Autodesk Fusion 360 part; units mm, degrees
(part 2 of 5)
sketch "Sketch1" plane through (0, 0, 0) normal (0, 0, 1) x (1, 0, 0)
  line L0 (-30.55, 69.6) -> (-28.55, 69.6)
  line L1 (-28.55, 69.6) -> (-28.55, 0)
  line L2 (-28.55, 0) -> (-30.55, 0)
  line L3 (-30.55, 0) -> (-30.55, 69.6)
  line L4 (28.55, 69.6) -> (30.55, 69.6)
  line L5 (30.55, 69.6) -> (30.55, 0)
  line L6 (30.55, 0) -> (28.55, 0)
  line L7 (28.55, 0) -> (28.55, 69.6)
  dimension "d1" = 69.6
  dimension "d2" = 69.6
  dimension "d3" = 2
  dimension "d4" = 2
  dimension "d5" = 57.1
  dimension "d6" = 28.55
  constraint horizontal L0
  constraint vertical L1
  constraint horizontal L2
  constraint vertical L3
  constraint horizontal L4
  constraint vertical L5
  constraint horizontal L6
  constraint vertical L7
  constraint horizontal L0.start L4.start
  constraint horizontal origin L1.end
  measures "d1" distance of L0 L2
  measures "d2" distance of L4 L6
  measures "d3" distance of L1 L3
  measures "d4" distance of L5 L7
  measures "d5" distance of L1 L7
  measures "d6" distance of origin L7
extrude "Extrude1" add sketch "Sketch1" along normal blind 20 makes body 1 at (-28.55, 46.4, 6.6667) makes body 2 at (30.55, 46.4, 6.6667)
sketch "Sketch3" plane through (0, 0, 20) normal (0, 0, 1) x (-1, 0, 0)
  line L0 (-28.55, 0) -> (-30.55, 0)
  line L1 (-30.55, 0) -> (-30.55, -69.6)
  line L2 (-30.55, -69.6) -> (-28.55, -69.6)
  line L3 (-28.55, -69.6) -> (-28.55, 0)
  arc A0 (-28.55, -69.6) -> (28.55, -69.6) centre (0, 38.699) ccw
  arc A1 (-30.55, -71.6) -> (30.55, -71.6) centre (0, 52.672) ccw
  line L4 (30.55, -71.6) -> (30.55, -69.6)
  line L5 (-30.55, -71.6) -> (-30.55, -69.6)
  line L6 (-28.55, -69.6) -> (-30.55, -69.6)
  line L7 (28.55, -69.6) -> (30.55, -69.6)
  point P0 (-28.55, -69.6)
  point P1 (28.55, -69.6)
  point P2 (0, -73.3)
  point P3 (0, -75.3)
  point P4 (30.55, -71.6)
  point P5 (-30.55, -71.6)
  point P6 (30.55, -69.6)
  dimension "d9" = 3.7
  dimension "d10" = 2
  dimension "d11" = 2
  dimension "d12" = 2
  constraint coincident P0 L2.end
  constraint coincident P2 A0
  constraint coincident P1 A0.end
  constraint vertical origin P2
  constraint vertical P2 P3
  constraint vertical L1.end P5
  constraint vertical P4 P6
  constraint coincident P3 A1
  constraint coincident P5 A1.start
  constraint coincident P4 A1.end
  constraint coincident P6 L4.end
  constraint coincident L1.end L2.start
  measures "d9" vertical distance of P0 P2
  measures "d10" distance of P2 P3
  measures "d11" distance of P4 P6
  measures "d12" distance of L1.end P5
extrude "Extrude2" add sketch "Sketch3" against normal blind 20 contours L2 A0 A1 L4 L5 L6 L7 bodies 1 2
sketch "Sketch4" plane through (30.55, 0, 0) normal (1, 0, 0) x (0, 1, 0)
  line L0 (0, 0) -> (71.6, 0)
  line L1 (71.6, 0) -> (71.6, 20)
  line L2 (71.6, 20) -> (0, 20)
  line L3 (0, 20) -> (0, 0)
  line L4 (0, 0) -> (20, 0)
  line L5 (20, 0) -> (20, -4)
  line L6 (20, -4) -> (0, -4)
  line L7 (0, -4) -> (0, 0)
  dimension "d15" = 4
  dimension "d16" = 20
  constraint horizontal L4
  constraint vertical L5
  constraint horizontal L6
  constraint vertical L7
  constraint coincident L0.start L3.end
  measures "d15" distance of L4 L6
  measures "d16" distance of L5 L7
extrude "Extrude3" add sketch "Sketch4" against normal blind 2 contours L0 L4 L5 L6 L7 bodies 1
sketch "Sketch5" plane through (-30.55, 0, 0) normal (-1, 0, 0) x (0, -1, 0)
  line L0 (-71.6, 0) -> (0, 0)
  line L1 (0, 0) -> (0, 20)
  line L2 (0, 20) -> (-71.6, 20)
  line L3 (-71.6, 20) -> (-71.6, 0)
  line L4 (0, 0) -> (-20, 0)
  line L5 (-20, 0) -> (-20, -4)
  line L6 (-20, -4) -> (0, -4)
  line L7 (0, -4) -> (0, 0)
  dimension "d19" = 4
  dimension "d20" = 20
  constraint horizontal L4
  constraint vertical L5
  constraint horizontal L6
  constraint vertical L7
  constraint coincident L0.end L1.start
  measures "d19" distance of L4 L6
  measures "d20" distance of L5 L7
extrude "Extrude4" add sketch "Sketch5" against normal blind 2 contours L0 L4 L5 L6 L7 bodies 1
fillet "Fillet2" radius 2 4 edges at (30.55, 71.6, 10) (-30.55, 71.6, 10) (29.55, 20, 0) (-29.55, 20, 0) on bodies 1
sketch "Sketch8" plane through (0, 0, 0) normal (0, -1, 0) x (1, 0, 0)
  line L0 (30.55, -4) -> (30.55, 20)
  line L1 (30.55, 20) -> (28.55, 20)
  line L2 (28.55, 20) -> (28.55, -4)
  line L3 (30.55, 20) -> (28.55, 20)
  line L4 (30.55, 36.5) -> (30.55, 20)
  line L5 (-30.55, 20) -> (-28.55, 20)
  line L6 (-30.55, 36.5) -> (-30.55, 20)
  line L7 (28.55, 20) -> (-28.55, 20)
  line L8 (-19.3, 36.5) -> (-19.3, 34.25)
  line L9 (-24.3, 29.25) -> (-26.05, 29.25)
  line L10 (19.3, 36.5) -> (19.3, 34.25)
  line L11 (24.3, 29.25) -> (26.05, 29.25)
  line L12 (-28.55, 26.75) -> (-28.55, 20)
  line L13 (28.55, 26.75) -> (28.55, 20)
  line L14 (-28.05, 39) -> (-21.8, 39)
  line L15 (21.8, 39) -> (28.05, 39)
  arc A0 (30.55, 36.5) -> (28.05, 39) centre (28.05, 36.5) ccw
  arc A1 (-28.05, 39) -> (-30.55, 36.5) centre (-28.05, 36.5) ccw
  arc A2 (21.8, 39) -> (19.3, 36.5) centre (21.8, 36.5) ccw
  arc A3 (28.55, 26.75) -> (26.05, 29.25) centre (26.05, 26.75) ccw
  arc A4 (-26.05, 29.25) -> (-28.55, 26.75) centre (-26.05, 26.75) ccw
  arc A5 (-19.3, 36.5) -> (-21.8, 39) centre (-21.8, 36.5) ccw
  arc A6 (19.3, 34.25) -> (24.3, 29.25) centre (24.3, 34.25) ccw
  arc A7 (-24.3, 29.25) -> (-19.3, 34.25) centre (-24.3, 34.25) ccw
  line L16 (28.55, -4) -> (30.55, -4)
  point P0 (-30.55, 39)
  point P1 (-19.3, 39)
  point P2 (-19.3, 29.25)
  point P3 (-28.55, 29.25)
  point P4 (19.3, 39)
  point P5 (19.3, 29.25)
  point P6 (28.55, 29.25)
  dimension "d41" = 61.1
  dimension "d51" = 9.75
  dimension "d52" = 9.75
  dimension "d53" = 9.25
  dimension "d54" = 9.25
  dimension "d55" = 11.25
  dimension "d56" = 9.25
  dimension "d57" = 2.5
  dimension "d58" = 2.5
  dimension "d59" = 5
  constraint horizontal L3
  constraint vertical L4
  constraint coincident L0.end L1.start
  constraint horizontal L5
  constraint vertical L6
  constraint horizontal L0.end L5.start
  constraint vertical L8
  constraint horizontal L9
  constraint vertical L10
  constraint horizontal L11
  constraint perpendicular L7 L12
  constraint coincident L1.end L2.start
  constraint perpendicular L3 L13
  constraint perpendicular L8 L14
  constraint horizontal P2 P5
  constraint tangent L15 A0
  constraint tangent L4 A0
  constraint coincident P0 L14
  constraint coincident P0 L6
  constraint tangent L14 A1
  constraint tangent L6 A1
  constraint equal A0 A1
  constraint coincident P4 L10
  constraint coincident P4 L15
  constraint tangent L10 A2
  constraint tangent L15 A2
  constraint coincident P6 L11
  constraint coincident P6 L13
  constraint tangent L11 A3
  constraint tangent L13 A3
  constraint equal A2 A3
  constraint coincident P3 L9
  constraint coincident P3 L12
  constraint tangent L9 A4
  constraint tangent L12 A4
  constraint equal A2 A4
  constraint coincident P1 L8
  constraint coincident P1 L14
  constraint tangent L8 A5
  constraint tangent L14 A5
  constraint equal A2 A5
  constraint coincident P5 L11
  constraint coincident P5 L10
  constraint tangent L11 A6
  constraint tangent L10 A6
  constraint coincident P2 L9
  constraint coincident P2 L8
  constraint tangent L9 A7
  constraint tangent L8 A7
  constraint equal A6 A7
  measures "d41" distance of L0.end L5.start
  measures "d51" distance of P1 P2
  measures "d52" distance of P4 P5
  measures "d53" distance of P2 P3
  measures "d54" distance of P5 P6
  measures "d55" distance of P0 P1
  measures "d56" distance of P6 L1.end
  measures "d57" radius of A0
  measures "d58" radius of A2
  measures "d59" radius of A6
extrude "Extrude6" add sketch "Sketch8" against normal blind 20 contours L1 L3 L4 L10 L11 L13 L15 A0 A2 A3 A6 | L5 L6 L8 L9 L12 L14 A1 A4 A5 A7 bodies 1
sketch "Sketch9" plane through (0, 20, 0) normal (0, 1, 0) x (-1, 0, 0)
  arc A0 (-19.3, 36.5) -> (-21.8, 39) centre (-21.8, 36.5) ccw
  line L0 (-21.8, 39) -> (-28.05, 39)
  arc A1 (-28.05, 39) -> (-30.55, 36.5) centre (-28.05, 36.5) ccw
  line L1 (-30.55, 36.5) -> (-30.55, 20)
  line L2 (-30.55, 20) -> (-28.55, 20)
  line L3 (-28.55, 20) -> (-28.55, 26.75)
  arc A2 (-26.05, 29.25) -> (-28.55, 26.75) centre (-26.05, 26.75) ccw
  line L4 (-26.05, 29.25) -> (-24.3, 29.25)
  arc A3 (-24.3, 29.25) -> (-19.3, 34.25) centre (-24.3, 34.25) ccw
  line L5 (-19.3, 34.25) -> (-19.3, 36.5)
  line L6 (30.55, 20) -> (30.55, 36.5)
  point P0 (-24.05, 34.05)
  point P1 (24.05, 34.05)
  dimension "d62" = 6.5
  dimension "d63" = 6.5
  dimension "d64" = 4.95
  constraint horizontal P0 P1
  measures "d62" distance of L1 P0
  measures "d63" distance of P1 L6
  measures "d64" distance of L0 P0
hole "Hole3" at (24.05, 20, 34.05) at (-24.05, 20, 34.05) direction (0, -1, 0) diameter 6.5 depth 12.5 tip angle 180 bodies 1
sketch "Sketch10" plane through (0, 7.5, 0) normal (0, 1, 0) x (-1, 0, 0)
  circle A0 centre (-24.05, 34.05) radius 3.25
  line L0 (-30.55, 36.5) -> (-30.55, 20)
  line L1 (30.55, 20) -> (30.55, 36.5)
  line L2 (-21.8, 39) -> (-28.05, 39)
  point P0 (-24.05, 34.05)
  point P1 (24.05, 34.05)
  dimension "d73" = 6.5
  dimension "d74" = 6.5
  dimension "d75" = 4.95
  constraint horizontal P0 P1
  measures "d73" distance of P0 L0
  measures "d74" distance of P1 L1
  measures "d75" distance of P0 L2
hole "Hole4" at (24.05, 7.5, 34.05) at (-24.05, 7.5, 34.05) direction (0, -1, 0) diameter 3.6 end through all counterbore diameter 6.5 counterbore depth 3 bodies 1
sketch "Sketch11" plane through (30.55, 0, 0) normal (1, 0, 0) x (0, 1, 0)
  line L0 (70.0221, 0) -> (70.0221, 20)
  line L1 (70.0221, 20) -> (20, 20)
  line L2 (20, 20) -> (20, 36.5)
  line L3 (20, 36.5) -> (0, 36.5)
  line L4 (0, 36.5) -> (0, -4)
  line L5 (20, -4) -> (20, -2)
  arc A0 (22, 0) -> (20, -2) centre (22, -2) ccw
  line L6 (22, 0) -> (70.0221, 0)
  arc A1 (8.659, 9.478) -> (8.6579, 10.5518) centre (7.8148, 10.014) ccw
  line L7 (8.659, 9.478) -> (3.8443, 1.8949)
  line L8 (3.8432, 18.1005) -> (8.6579, 10.5518)
  line L9 (0.0001, 36.7902) -> (0.0001, -5.2598)
  arc A2 (3.8432, 18.1005) -> (2.0001, 17.5628) centre (3.0001, 17.5628) ccw
  arc A3 (2.0001, 2.4309) -> (3.8443, 1.8949) centre (3.0001, 2.4309) ccw
  arc A4 (18.0001, 17.5628) -> (16.157, 18.1005) centre (17.0001, 17.5628) ccw
  line L10 (16.088, 20.7084) -> (10.853, 12.3732)
  line L11 (9.1559, 12.3786) -> (3.9952, 20.7138)
  line L12 (3.99, -0.735) -> (9.1549, 7.6441)
  line L13 (15.2412, 22.2402) -> (4.8454, 22.2402)
  line L14 (2.0001, 17.5628) -> (2.0001, 2.4309)
  arc A5 (10.8541, 7.6495) -> (9.1549, 7.6441) centre (10.0062, 7.1193) ccw
  line L15 (20.0001, 40.5402) -> (0.0001, 40.5402)
  arc A6 (3.99, -0.735) -> (4.8412, -2.2598) centre (4.8412, -1.2598) ccw
  line L16 (20.0001, 36.7902) -> (0.0001, 36.7902)
  arc A7 (4.8454, 22.2402) -> (3.9952, 20.7138) centre (4.8454, 21.2402) ccw
  line L17 (15.2454, -2.2598) -> (4.8412, -2.2598)
  line L18 (18.0001, 17.5628) -> (18.0001, 2.4309)
  arc A8 (16.088, 20.7084) -> (15.2412, 22.2402) centre (15.2412, 21.2402) ccw
  line L19 (16.1559, 1.8949) -> (11.3412, 9.478)
  arc A9 (9.1559, 12.3786) -> (10.853, 12.3732) centre (10.0062, 12.9051) ccw
  line L20 (10.8541, 7.6495) -> (16.0933, -0.7296)
  line L21 (11.3423, 10.5518) -> (16.157, 18.1005)
  arc A10 (11.3423, 10.5518) -> (11.3412, 9.478) centre (12.1854, 10.014) ccw
  line L22 (12.713, -5.2598) -> (20.0001, -5.2598)
  arc A11 (16.1559, 1.8949) -> (18.0001, 2.4309) centre (17.0001, 2.4309) ccw
  arc A12 (15.2454, -2.2598) -> (16.0933, -0.7296) centre (15.2454, -1.2598) ccw
  line L23 (0.0001, -5.2598) -> (7.2872, -5.2598)
  line L24 (20.0001, -5.2598) -> (20.0001, 36.7902)
  line L25 (0, -4) -> (20, -4)
  point P0 (9.0001, 11.2652)
  point P1 (11.0001, 11.2652)
  point P2 (18.0001, -1.0098)
  point P3 (2.0001, 20.9902)
  point P4 (10.0001, 10.2652)
  point P5 (10.0062, 10.014)
  point P6 (17.0501, 22.2402)
  point P7 (2.0001, -1.0098)
  point P8 (3.0501, -2.2598)
  point P9 (17.0501, -2.2598)
  point P10 (3.0501, 22.2402)
  point P11 (10.0001, 12.2652)
  point P12 (0.0001, 12.2652)
  point P13 (18.0001, 20.9902)
  dimension "d82" = 2
  dimension "d83" = 2
  dimension "d86" = 22
  dimension "d87" = 22
  dimension "d88" = 14
  dimension "d89" = 14
  dimension "d91" = 3.05
  dimension "d92" = 1
  dimension "d150" = 24.5
  dimension "d151" = 5.7857
  dimension "d152" = 18.3
  constraint perpendicular L13 L24
  constraint perpendicular L13 L14
  constraint coincident P6 L10
  constraint coincident P6 L13
  constraint tangent L10 A8
  constraint tangent L13 A8
  constraint coincident P10 L13
  constraint coincident P10 L11
  constraint tangent L13 A7
  constraint tangent L11 A7
  constraint equal A7 A8
  constraint tangent L11 A9
  constraint tangent L10 A9
  constraint equal A8 A9
  constraint tangent A1 L8
  constraint tangent A1 L7
  constraint equal A1 A8
  constraint coincident P7 L7
  constraint coincident P7 L14
  constraint tangent L7 A3
  constraint tangent A3 L14
  constraint equal A3 A8
  constraint coincident P3 L14
  constraint coincident P3 L8
  constraint tangent A2 L14
  constraint tangent L8 A2
  constraint equal A2 A8
  constraint coincident P8 L12
  constraint coincident P8 L17
  constraint tangent L12 A6
  constraint tangent A6 L17
  constraint equal A6 A8
  constraint coincident P9 L17
  constraint coincident P9 L20
  constraint tangent L17 A12
  constraint tangent L20 A12
  constraint equal A8 A12
  constraint coincident P2 L19
  constraint coincident P2 L18
  constraint tangent L19 A11
  constraint tangent L18 A11
  constraint equal A8 A11
  constraint coincident P13 L21
  constraint coincident P13 L18
  constraint tangent A4 L21
  constraint tangent A4 L18
  constraint equal A4 A8
  constraint tangent L19 A10
  constraint tangent L21 A10
  constraint equal A8 A10
  constraint tangent L12 A5
  constraint tangent A5 L20
  constraint equal A5 A8
  constraint vertical A9.centre A5.centre
  constraint horizontal A10.centre A1.centre
  constraint horizontal A10.centre P5
  constraint vertical A5.centre P5
  measures "d82" distance of L18 L24
  measures "d83" distance of L9 L14
  measures "d86" distance of P2 P13
  measures "d87" distance of P3 P7
  measures "d88" distance of P8 P9
  measures "d89" distance of P6 P10
  measures "d91" distance of P8 L9
  measures "d92" radius of A8
  measures "d150" distance of L13 L17
  measures "d151" distance of A9.centre A5.centre
  measures "d152" distance of L13 L15
extrude "Extrude7" cut sketch "Sketch11" against normal blind 65 contours A1 L7 L8 A2 A3 L14 | A4 L18 L19 L21 A10 A11 | L10 L11 L13 A7 A8 A9 | L12 A5 A6 L17 L20 A12 bodies 1
sketch "Sketch12" plane through (30.55, 0, 0) normal (1, 0, 0) x (0, 1, 0)
  line L0 (16.1559, 1.8949) -> (11.3412, 9.478)
  arc A0 (11.3423, 10.5518) -> (11.3412, 9.478) centre (12.1854, 10.014) ccw
  line L1 (11.3423, 10.5518) -> (16.157, 18.1005)
  arc A1 (18.0001, 17.5628) -> (16.157, 18.1005) centre (17.0001, 17.5628) ccw
  line L2 (18.0001, 17.5628) -> (18.0001, 2.4309)
  arc A2 (16.1559, 1.8949) -> (18.0001, 2.4309) centre (17.0001, 2.4309) ccw
  line L3 (15.2454, -2.2598) -> (4.8412, -2.2598)
  arc A3 (3.99, -0.735) -> (4.8412, -2.2598) centre (4.8412, -1.2598) ccw
  line L4 (3.99, -0.735) -> (9.1549, 7.6441)
  arc A4 (10.8541, 7.6495) -> (9.1549, 7.6441) centre (10.0062, 7.1193) ccw
  line L5 (10.8541, 7.6495) -> (16.0933, -0.7296)
  arc A5 (15.2454, -2.2598) -> (16.0933, -0.7296) centre (15.2454, -1.2598) ccw
  line L6 (4.8454, 22.2402) -> (15.2412, 22.2402)
  arc A6 (16.088, 20.7084) -> (15.2412, 22.2402) centre (15.2412, 21.2402) ccw
  line L7 (16.088, 20.7084) -> (10.853, 12.3732)
  arc A7 (9.1559, 12.3786) -> (10.853, 12.3732) centre (10.0062, 12.9051) ccw
  line L8 (9.1559, 12.3786) -> (3.9952, 20.7138)
  arc A8 (4.8454, 22.2402) -> (3.9952, 20.7138) centre (4.8454, 21.2402) ccw
  line L9 (2.0001, 2.4309) -> (2.0001, 17.5628)
  arc A9 (3.8432, 18.1005) -> (2.0001, 17.5628) centre (3.0001, 17.5628) ccw
  line L10 (3.8432, 18.1005) -> (8.6579, 10.5518)
  arc A10 (8.659, 9.478) -> (8.6579, 10.5518) centre (7.8148, 10.014) ccw
  line L11 (8.659, 9.478) -> (3.8443, 1.8949)
  arc A11 (2.0001, 2.4309) -> (3.8443, 1.8949) centre (3.0001, 2.4309) ccw
  line L12 (70.0221, 0) -> (70.0221, 20)
  line L13 (70.0221, 20) -> (20, 20)
  line L14 (20, 20) -> (20, 36.5)
  line L15 (20, 36.5) -> (0, 36.5)
  line L16 (0, 36.5) -> (0, -4)
  line L17 (20, -4) -> (20, -2)
  arc A12 (22, 0) -> (20, -2) centre (22, -2) ccw
  line L18 (22, 0) -> (70.0221, 0)
  line L19 (27.57, 18) -> (62.43, 18)
  line L20 (68, 14.6743) -> (68, 5.3257)
  line L21 (62.43, 2) -> (27.57, 2)
  line L22 (22, 5.3257) -> (22, 14.6743)
  line L23 (27.4327, 17.0192) -> (44.7253, 12.0785)
  line L24 (45.2747, 12.0785) -> (62.5673, 17.0192)
  line L25 (66.7253, 15.6358) -> (48.6827, 10.4808)
  line L26 (48.6827, 9.5192) -> (66.7253, 4.3642)
  line L27 (62.5673, 2.9808) -> (45.2747, 7.9215)
  line L28 (44.7253, 7.9215) -> (27.4327, 2.9808)
  line L29 (23.2747, 4.3642) -> (41.3173, 9.5192)
  line L30 (41.3173, 10.4808) -> (23.2747, 15.6358)
  arc A13 (23.2747, 15.6358) -> (22, 14.6743) centre (23, 14.6743) ccw
  arc A14 (22, 5.3257) -> (23.2747, 4.3642) centre (23, 5.3257) ccw
  arc A15 (66.7253, 4.3642) -> (68, 5.3257) centre (67, 5.3257) ccw
  arc A16 (68, 14.6743) -> (66.7253, 15.6358) centre (67, 14.6743) ccw
  arc A17 (41.3173, 9.5192) -> (41.3173, 10.4808) centre (41.18, 10) ccw
  arc A18 (48.6827, 10.4808) -> (48.6827, 9.5192) centre (48.82, 10) ccw
  arc A19 (27.4327, 2.9808) -> (27.57, 2) centre (27.57, 2.5) ccw
  arc A20 (62.43, 2) -> (62.5673, 2.9808) centre (62.43, 2.5) ccw
  arc A21 (62.5673, 17.0192) -> (62.43, 18) centre (62.43, 17.5) ccw
  arc A22 (27.57, 18) -> (27.4327, 17.0192) centre (27.57, 17.5) ccw
  arc A23 (44.7253, 12.0785) -> (45.2747, 12.0785) centre (45, 13.04) ccw
  arc A24 (45.2747, 7.9215) -> (44.7253, 7.9215) centre (45, 6.96) ccw
  line L31 (0, -4) -> (20, -4)
  point P0 (24, 18)
  point P1 (22, 16)
  point P2 (22, 4)
  point P3 (24, 2)
  point P4 (66, 18)
  point P5 (68, 16)
  point P6 (68, 4)
  point P7 (66, 2)
  point P8 (45, 10)
  point P9 (45, 12)
  point P10 (43, 10)
  point P11 (45, 8)
  point P12 (47, 10)
  dimension "d95" = 1
  dimension "d96" = 0.5
  dimension "d97" = 0.5
  dimension "d98" = 1
  constraint horizontal L19
  constraint vertical L20
  constraint horizontal L21
  constraint vertical L22
  constraint coincident L19 P0
  constraint coincident L22 P1
  constraint coincident L22 P2
  constraint coincident L21 P3
  constraint coincident L19 P4
  constraint coincident L20 P5
  constraint coincident L20 P6
  constraint coincident L21 P7
  constraint parallel L24 L25
  constraint parallel L23 L26
  constraint parallel L26 L27
  constraint parallel L25 L28
  constraint parallel L28 L29
  constraint parallel L27 L30
  constraint tangent L30 A13
  constraint tangent L22 A13
  constraint tangent L29 A14
  constraint tangent L22 A14
  constraint equal A13 A14
  constraint tangent L26 A15
  constraint tangent L20 A15
  constraint equal A13 A15
  constraint tangent L25 A16
  constraint tangent L20 A16
  constraint equal A13 A16
  constraint tangent L30 A17
  constraint tangent L29 A17
  constraint tangent L26 A18
  constraint tangent L25 A18
  constraint equal A17 A18
  constraint tangent L28 A19
  constraint tangent L21 A19
  constraint tangent L21 A20
  constraint tangent L27 A20
  constraint equal A19 A20
  constraint tangent L24 A21
  constraint tangent L19 A21
  constraint equal A19 A21
  constraint tangent L23 A22
  constraint tangent L19 A22
  constraint equal A19 A22
  constraint tangent L23 A23
  constraint tangent L24 A23
  constraint tangent L28 A24
  constraint tangent L27 A24
  constraint equal A23 A24
  measures "d95" radius of A13
  measures "d96" radius of A17
  measures "d97" radius of A19
  measures "d98" radius of A23
extrude "Extrude8" cut sketch "Sketch12" against normal blind 65 contours L19 L23 L24 A21 A22 A23 | L20 L25 L26 A15 A16 A18 | L21 L27 L28 A19 A20 A24 | L22 L29 L30 A13 A14 A17 bodies 1
sketch "Sketch15" plane through (0, 0, 0) normal (0, -1, 0) x (1, 0, 0)
  circle A0 centre (-24.05, 34.05) radius 1.8
  line L0 (-28.55, -4) -> (-28.55, 26.75)
  arc A1 (-26.05, 29.25) -> (-28.55, 26.75) centre (-26.05, 26.75) ccw
  line L1 (-26.05, 29.25) -> (-24.3, 29.25)
  arc A2 (-24.3, 29.25) -> (-19.3, 34.25) centre (-24.3, 34.25) ccw
  line L2 (-19.3, 34.25) -> (-19.3, 36.5)
  arc A3 (-19.3, 36.5) -> (-21.8, 39) centre (-21.8, 36.5) ccw
  line L3 (-21.8, 39) -> (-28.05, 39)
  arc A4 (-28.05, 39) -> (-30.55, 36.5) centre (-28.05, 36.5) ccw
  line L4 (-30.55, 36.5) -> (-30.55, -4)
  line L5 (-21.4029, 18) -> (21.4029, 18)
  line L6 (26.55, 15.2137) -> (26.55, 4.7863)
  line L7 (21.4029, 2) -> (-21.4029, 2)
  line L8 (-26.55, 4.7863) -> (-26.55, 15.2137)
  line L9 (28.55, 0) -> (-28.55, 0)
  line L10 (28.55, 20) -> (-28.55, 20)
  line L11 (28.55, -4) -> (28.55, 26.75)
  line L12 (-21.527, 2.9844) -> (-1.241, 8.182)
  line L13 (1.241, 8.182) -> (21.527, 2.9844)
  line L14 (25.3035, 3.8171) -> (3.8571, 9.2732)
  line L15 (3.8571, 10.7268) -> (25.3035, 16.1829)
  line L16 (21.527, 17.0156) -> (1.241, 11.818)
  line L17 (-1.241, 11.818) -> (-21.527, 17.0156)
  line L18 (-25.3035, 16.1829) -> (-3.8571, 10.7268)
  line L19 (-3.8571, 9.2732) -> (-25.3035, 3.8171)
  arc A5 (-25.3035, 16.1829) -> (-26.55, 15.2137) centre (-25.55, 15.2137) ccw
  arc A6 (-26.55, 4.7863) -> (-25.3035, 3.8171) centre (-25.55, 4.7863) ccw
  arc A7 (25.3035, 3.8171) -> (26.55, 4.7863) centre (25.55, 4.7863) ccw
  arc A8 (26.55, 15.2137) -> (25.3035, 16.1829) centre (25.55, 15.2137) ccw
  arc A9 (-3.8571, 9.2732) -> (-3.8571, 10.7268) centre (-4.042, 10) ccw
  arc A10 (3.8571, 10.7268) -> (3.8571, 9.2732) centre (4.042, 10) ccw
  arc A11 (-21.527, 2.9844) -> (-21.4029, 2) centre (-21.4029, 2.5) ccw
  arc A12 (21.4029, 2) -> (21.527, 2.9844) centre (21.4029, 2.5) ccw
  arc A13 (21.527, 17.0156) -> (21.4029, 18) centre (21.4029, 17.5) ccw
  arc A14 (-21.4029, 18) -> (-21.527, 17.0156) centre (-21.4029, 17.5) ccw
  arc A15 (-1.241, 11.818) -> (1.241, 11.818) centre (0, 16.6615) ccw
  arc A16 (1.241, 8.182) -> (-1.241, 8.182) centre (0, 3.3385) ccw
  line L20 (-30.55, -4) -> (-28.55, -4)
  point P0 (-26.55, 18)
  point P1 (26.55, 18)
  point P2 (26.55, 2)
  point P3 (-25.05, 18)
  point P4 (-25.05, 2)
  point P5 (25.05, 18)
  point P6 (25.05, 2)
  point P7 (0, 10)
  point P8 (-26.55, 16.5)
  point P9 (-26.55, 3.5)
  point P10 (26.55, 16.5)
  point P11 (26.55, 3.5)
  point P12 (0, 8.5)
  point P13 (-1, 10)
  point P14 (0, 11.5)
  point P15 (1, 10)
  dimension "d102" = 2
  dimension "d103" = 2
  dimension "d104" = 2
  dimension "d105" = 2
  dimension "d106" = 1.5
  dimension "d107" = 1.5
  dimension "d108" = 1.5
  dimension "d109" = 1.5
  dimension "d110" = 26.55
  dimension "d112" = 1
  dimension "d113" = 0.75
  dimension "d114" = 0.5
  dimension "d115" = 3
  dimension "d117" = 1.5
  dimension "d118" = 5
  constraint horizontal L5
  constraint vertical L6
  constraint horizontal L7
  constraint vertical L8
  constraint coincident L5 P3
  constraint coincident L7 P4
  constraint coincident L5 P5
  constraint coincident L7 P6
  constraint coincident L8 P8
  constraint coincident L8 P9
  constraint coincident L6 P10
  constraint coincident L6 P11
  constraint vertical P3 P4
  constraint horizontal P8 P10
  constraint horizontal P9 P11
  constraint vertical P5 P6
  constraint coincident P0 L8
  constraint tangent L18 A5
  constraint tangent L8 A5
  constraint tangent L19 A6
  constraint tangent L8 A6
  constraint equal A5 A6
  constraint coincident P2 L6
  constraint tangent L14 A7
  constraint tangent L6 A7
  constraint equal A5 A7
  constraint coincident P1 L6
  constraint tangent L6 A8
  constraint tangent L15 A8
  constraint equal A5 A8
  constraint tangent L19 A9
  constraint tangent L18 A9
  constraint tangent L14 A10
  constraint tangent L15 A10
  constraint equal A9 A10
  constraint tangent L12 A11
  constraint tangent L7 A11
  constraint coincident P2 L7
  constraint tangent L13 A12
  constraint tangent L7 A12
  constraint equal A11 A12
  constraint coincident P1 L5
  constraint tangent L16 A13
  constraint tangent L5 A13
  constraint equal A11 A13
  constraint coincident P0 L5
  constraint tangent L17 A14
  constraint tangent L5 A14
  constraint equal A11 A14
  constraint vertical P12 P14
  constraint horizontal A9.centre A10.centre
  constraint vertical P7 P12
  constraint horizontal P7 A10.centre
  constraint tangent L17 A15
  constraint tangent L16 A15
  constraint tangent L12 A16
  constraint tangent L13 A16
  constraint equal A15 A16
  measures "d102" distance of L0 L8
  measures "d103" distance of L7 L9
  measures "d104" distance of L5 L10
  measures "d105" distance of L6 L11
  measures "d106" distance of P0 P3
  measures "d107" distance of P0 P8
  measures "d108" distance of P1 P5
  measures "d109" distance of P2 P11
  measures "d110" horizontal distance of P0 P7
  measures "d112" radius of A5
  measures "d113" radius of A9
  measures "d114" radius of A11
  measures "d115" distance of P12 P14
  measures "d117" distance of P7 P12
  measures "d118" radius of A15
extrude "Extrude9" cut sketch "Sketch15" against normal blind 80 contours L5 L16 L17 A13 A14 A15 | L6 L14 L15 A7 A8 A10 | L7 L12 L13 A11 A12 A16 | L8 L18 L19 A5 A6 A9 bodies 1
sketch "Sketch17" plane through (0, 0, 0) normal (0, -1, 0) x (1, 0, 0)
  circle A0 centre (24.05, 34.05) radius 1.8
  line L0 (30.55, -4) -> (30.55, 36.5)
  arc A1 (30.55, 36.5) -> (28.05, 39) centre (28.05, 36.5) ccw
  line L1 (28.05, 39) -> (21.8, 39)
  arc A2 (21.8, 39) -> (19.3, 36.5) centre (21.8, 36.5) ccw
  line L2 (19.3, 36.5) -> (19.3, 34.25)
  arc A3 (19.3, 34.25) -> (24.3, 29.25) centre (24.3, 34.25) ccw
  line L3 (24.3, 29.25) -> (26.05, 29.25)
  arc A4 (28.55, 26.75) -> (26.05, 29.25) centre (26.05, 26.75) ccw
  line L4 (28.55, 26.75) -> (28.55, -4)
  line L5 (28.55, -4) -> (30.55, -4)
  line L6 (28.55, -4) -> (30.55, -4)
  line L7 (30.55, -4) -> (30.55, -18.55)
  line L8 (30.55, -18.55) -> (28.55, -18.55)
  line L9 (28.55, -18.55) -> (28.55, -4)
  line L10 (-28.55, -4) -> (-30.55, -4)
  line L11 (-30.55, -4) -> (-30.55, -18.55)
  line L12 (-30.55, -18.55) -> (-28.55, -18.55)
  line L13 (-28.55, -18.55) -> (-28.55, -4)
  line L14 (-30.55, -18.55) -> (-40.55, -18.55)
  line L15 (-40.55, -18.55) -> (-40.55, -16.05)
  line L16 (-40.55, -16.05) -> (-30.55, -16.05)
  line L17 (-30.55, -16.05) -> (-30.55, -18.55)
  line L18 (30.55, -18.55) -> (40.55, -18.55)
  line L19 (40.55, -18.55) -> (40.55, -16.05)
  line L20 (40.55, -16.05) -> (30.55, -16.05)
  line L21 (30.55, -16.05) -> (30.55, -18.55)
  dimension "d128" = 57.55
  dimension "d129" = 57.1
  dimension "d130" = 2
  dimension "d131" = 2
  dimension "d132" = 2.5
  dimension "d133" = 10
  dimension "d134" = 10
  dimension "d135" = 2.5
  constraint horizontal L6
  constraint vertical L7
  constraint horizontal L8
  constraint vertical L9
  constraint coincident L4.end L5.start
  constraint horizontal L10
  constraint vertical L11
  constraint horizontal L12
  constraint vertical L13
  constraint horizontal L7.end L12.end
  constraint horizontal L4.end L10.start
  constraint horizontal L14
  constraint vertical L15
  constraint horizontal L16
  constraint vertical L17
  constraint horizontal L18
  constraint vertical L19
  constraint horizontal L20
  constraint vertical L21
  measures "d128" distance of L1 L8
  measures "d129" distance of L9 L13
  measures "d130" distance of L11 L13
  measures "d131" distance of L7 L9
  measures "d132" distance of L18 L20
  measures "d133" distance of L7 L19
  measures "d134" distance of L15 L17
  measures "d135" distance of L14 L16
extrude "Extrude11" add sketch "Sketch17" against normal blind 20 contours L5 L6 L7 L8 L9 L21 | L7 L18 L19 L20 L21 | L10 L11 L12 L13 L17 | L11 L14 L15 L16 L17 bodies 1
fillet "Fillet3" radius 2 2 edges at (40.55, 20, -17.3) (-40.55, 20, -17.3) on bodies 1
fillet "Fillet4" radius 2 2 edges at (-29.55, 20, 20) (29.55, 20, 20) on bodies 1
extrude "Extrude12" cut 2 faces at (-32.55, 12.6667, -18.55) (32.55, 12.6667, -18.55) along direction (0, 0, 1) blind 0.05 on bodies 1 bodies 1
extrude "Extrude13" add 2 faces at (33.8833, 12.6667, -16.05) (-33.8833, 12.6667, -16.05) along direction (0, 0, 1) blind 7.55 on bodies 1 bodies 1
sketch "Sketch19" plane through (0, 0, -8.5) normal (0, 0, 1) x (-1, 0, 0)
  arc A0 (-40.55, -18) -> (-38.55, -20) centre (-38.55, -18) ccw
  line L0 (-38.55, -20) -> (-30.55, -20)
  line L1 (-30.55, -20) -> (-30.55, 0)
  line L2 (-30.55, 0) -> (-40.55, 0)
  line L3 (-40.55, 0) -> (-40.55, -18)
  point P0 (-34.75, -10)
  point P1 (34.75, -10)
  dimension "d159" = 69.5
  dimension "d160" = 5.8
  dimension "d161" = 10
  constraint horizontal P0 P1
  measures "d159" distance of P0 P1
  measures "d160" distance of L3 P0
  measures "d161" distance of L2 P0
hole "Hole6" at (-34.75, 10, -8.5) at (34.75, 10, -8.5) direction (0, 0, -1) diameter 5.3 depth 10 tip angle 118 counterbore diameter 10 counterbore depth 5 bodies 1
sketch "Sketch20" plane through (0, 0, -8.5) normal (0, 0, 1) x (-1, 0, 0)
  arc A0 (-30.55, -7.2871) -> (-30.55, -12.7129) centre (-34.75, -10) ccw
  line L0 (-30.55, -7.2871) -> (-30.55, 0)
  line L1 (-30.55, 0) -> (-40.55, 0)
  line L2 (-40.55, 0) -> (-40.55, -18)
  arc A1 (-40.55, -18) -> (-38.55, -20) centre (-38.55, -18) ccw
  line L3 (-38.55, -20) -> (-30.55, -20)
  line L4 (-30.55, -20) -> (-30.55, -12.7129)
  circle A2 centre (-34.75, -10) radius 5
  circle A3 centre (34.75, -10) radius 5
  dimension "d167" = 10
  dimension "d168" = 10
  dimension "d169" = 69.5
  constraint concentric A0 A2
  constraint horizontal A0.centre A3.centre
  measures "d167" diameter of A2
  measures "d168" diameter of A3
  measures "d169" distance of A0.centre A3.centre
extrude "Extrude14" cut sketch "Sketch20" along normal blind 7 contours A0 A2 | A3 bodies 1
equation "d6 = ( 57.1 / 2 ) * 1 mm"
equation "d64 = 6.5 mm - 1.55 mm"
equation "d75 = 6.5 mm - 1.55 mm"
equation "d110 = ( 53.1 / 2 ) * 1 mm"
equation "d157 = 10 mm - 2.45 mm"

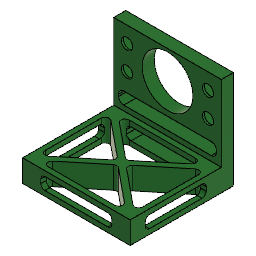
design "LGR Height Extension"
Autodesk Fusion 360 part; units mm, degrees
sketch "Sketch1" plane through (0, 0, 0) normal (0, 0, 1) x (1, 0, 0)
  line L0 (-28.575, 22.5) -> (28.575, 22.5)
  line L1 (28.575, 22.5) -> (28.575, -22.5)
  line L2 (28.575, -22.5) -> (-28.575, -22.5)
  line L3 (-28.575, -22.5) -> (-28.575, 22.5)
  dimension "d1" = 45
  dimension "d2" = 57.15
  dimension "d7" = 28.575
  dimension "d8" = 22.5
  constraint horizontal L0
  constraint vertical L1
  constraint horizontal L2
  constraint vertical L3
  measures "d1" distance of L0 L2
  measures "d2" distance of L1 L3
  measures "d7" distance of origin L1
  measures "d8" distance of origin L0
extrude "Extrude1" add sketch "Sketch1" along normal blind 1 makes body 1
sketch "Sketch3" plane through (0, 0, 1) normal (0, 0, 1) x (-1, 0, 0)
  line L0 (28.575, 22.5) -> (-28.575, 22.5)
  line L1 (-28.575, 22.5) -> (-28.575, -22.5)
  line L2 (-28.575, -22.5) -> (28.575, -22.5)
  line L3 (28.575, -22.5) -> (28.575, 22.5)
  line L4 (28.575, -22.5) -> (-28.575, -22.5)
  line L5 (-28.575, -22.5) -> (-28.575, -23.5)
  line L6 (-28.575, -23.5) -> (28.575, -23.5)
  line L7 (28.575, -23.5) -> (28.575, -22.5)
  dimension "d9" = 1
  dimension "d10" = 57.15
  constraint horizontal L4
  constraint vertical L5
  constraint horizontal L6
  constraint vertical L7
  constraint coincident L2.end L3.start
  measures "d9" distance of L4 L6
  measures "d10" distance of L5 L7
extrude "Extrude2" add sketch "Sketch3" along normal blind 45 separate body contours L2 L4 L5 L6 L7 makes body 2
extrude "Extrude3" add 1 faces at (-9.525, 23.1667, 1) along direction (0, 0, -1) blind 1 on bodies 2 bodies 1 2
extrude "Extrude4" add 1 faces at (9.525, 23.5, 30.6667) along direction (0, 1, 0) blind 5 on bodies 1 bodies 1
extrude "Extrude5" add 1 faces at (-9.525, 11.5, 0) along direction (0, 0, -1) blind 5 on bodies 1 bodies 1
sketch "Sketch5" plane through (0, 28.5, 0) normal (0, 1, 0) x (-1, 0, 0)
  line L0 (28.575, -5) -> (28.575, 46)
  line L1 (28.575, 46) -> (-28.575, 46)
  line L2 (-28.575, 46) -> (-28.575, -5)
  line L3 (-28.575, -5) -> (28.575, -5)
  point P0 (-20, 30.5)
  point P1 (20, 30.5)
  point P2 (-20, 18.5)
  point P3 (20, 18.5)
  dimension "d28" = 40
  dimension "d29" = 12
  dimension "d31" = 8.575
  dimension "d38" = 23.5
  constraint horizontal P0 P1
  constraint vertical P1 P3
  constraint horizontal P2 P3
  constraint vertical P0 P2
  measures "d28" distance of P0 P1
  measures "d29" distance of P1 P3
  measures "d31" distance of L2 P0
  measures "d38" distance of L3 P2
hole "Hole2" at (20, 28.5, 30.5) at (-20, 28.5, 30.5) at (-20, 28.5, 18.5) at (20, 28.5, 18.5) direction (0, -1, 0) diameter 5.5 depth 6 tip angle 180 counterbore diameter 10 counterbore depth 5 bodies 1
extrude "Extrude6" cut 1 faces at (-28.575, 9.5, -3) along direction (-1, 0, 0) blind 0 and the other way blind 2 on bodies 1 bodies 1
extrude "Extrude7" cut 1 faces at (28.575, 9.5, -3) along direction (1, 0, 0) blind 0 and the other way blind 2 on bodies 1 bodies 1
extrude "Extrude8" cut 1 faces at (-8.8583, 24.5, 46) along direction (0, 0, 1) blind 0 and the other way blind 7.5 on bodies 1 bodies 1
sketch "Sketch6" plane through (0, 28.5, 0) normal (0, 1, 0) x (-1, 0, 0)
  line L0 (26.575, 38.5) -> (-26.575, 38.5)
  line L1 (-26.575, 38.5) -> (-26.575, -5)
  line L2 (-26.575, -5) -> (26.575, -5)
  line L3 (26.575, -5) -> (26.575, 38.5)
  circle A0 centre (20, 18.5) radius 5
  circle A1 centre (-20, 30.5) radius 5
  circle A2 centre (20, 30.5) radius 5
  circle A3 centre (-20, 18.5) radius 5
  circle A4 centre (0, 24.5) radius 12.5
  dimension "d51" = 25
  dimension "d52" = 20
  dimension "d53" = 6
  measures "d51" diameter of A4
  measures "d52" horizontal distance of A3.centre A4.centre
  measures "d53" vertical distance of A2.centre A4.centre
extrude "Extrude9" cut sketch "Sketch6" along normal blind 0 and the other way blind 6 contours A4 bodies 1
sketch "Sketch9" plane through (0, 0, 1) normal (0, 0, 1) x (-1, 0, 0)
  line L0 (-26.575, 22.5) -> (-26.575, -22.5)
  line L1 (-26.575, -22.5) -> (26.575, -22.5)
  line L2 (26.575, -22.5) -> (26.575, 22.5)
  line L3 (26.575, 22.5) -> (-26.575, 22.5)
  line L4 (16.3972, -20) -> (-16.3972, -20)
  line L5 (24.075, -13.7886) -> (24.075, 13.7886)
  line L6 (16.3972, 20) -> (-16.3972, 20)
  line L7 (-24.075, 13.7886) -> (-24.075, -13.7886)
  line L8 (-1.2665, -3.0362) -> (-17.6637, -16.4521)
  line L9 (1.2665, -3.0362) -> (17.6637, -16.4521)
  line L10 (20.8111, -15.3386) -> (3.9009, -1.55)
  line L11 (3.9009, 1.55) -> (20.8111, 15.3386)
  line L12 (17.6637, 16.4521) -> (1.2665, 3.0362)
  line L13 (-1.2665, 3.0362) -> (-17.6637, 16.4521)
  line L14 (-20.8111, 15.3386) -> (-3.9009, 1.55)
  line L15 (-3.9009, -1.55) -> (-20.8111, -15.3386)
  arc A0 (20.8111, -15.3386) -> (24.075, -13.7886) centre (22.075, -13.7886) ccw
  arc A1 (3.9009, 1.55) -> (3.9009, -1.55) centre (5.1648, 0) ccw
  arc A2 (24.075, 13.7886) -> (20.8111, 15.3386) centre (22.075, 13.7886) ccw
  arc A3 (17.6637, 16.4521) -> (16.3972, 20) centre (16.3972, 18) ccw
  arc A4 (-16.3972, 20) -> (-17.6637, 16.4521) centre (-16.3972, 18) ccw
  arc A5 (-1.2665, 3.0362) -> (1.2665, 3.0362) centre (0, 4.5841) ccw
  arc A6 (-3.9009, -1.55) -> (-3.9009, 1.55) centre (-5.1648, 0) ccw
  arc A7 (-20.8111, 15.3386) -> (-24.075, 13.7886) centre (-22.075, 13.7886) ccw
  arc A8 (-24.075, -13.7886) -> (-20.8111, -15.3386) centre (-22.075, -13.7886) ccw
  arc A9 (-17.6637, -16.4521) -> (-16.3972, -20) centre (-16.3972, -18) ccw
  arc A10 (16.3972, -20) -> (17.6637, -16.4521) centre (16.3972, -18) ccw
  arc A11 (1.2665, -3.0362) -> (-1.2665, -3.0362) centre (0, -4.5841) ccw
  point P0 (22, -20)
  point P1 (-22, -20)
  point P2 (24.075, -18)
  point P3 (24.075, 18)
  point P4 (22, 20)
  point P5 (-22, 20)
  point P6 (-24.075, 18)
  point P7 (-24.075, -18)
  point P8 (0, -2)
  point P9 (-2, 0)
  point P10 (0, 2)
  point P11 (2, 0)
  dimension "d93" = 44
  dimension "d94" = 44
  dimension "d95" = 36
  dimension "d96" = 36
  dimension "d97" = 22
  dimension "d98" = 22
  dimension "d99" = 18
  dimension "d100" = 18
  dimension "d101" = 2.5
  dimension "d102" = 2.5
  dimension "d103" = 2.5
  dimension "d104" = 2.5
  dimension "d105" = 2
  dimension "d112" = 2
  constraint horizontal L4
  constraint parallel L2 L5
  constraint horizontal L6
  constraint parallel L0 L7
  constraint coincident P2 L10
  constraint coincident P2 L5
  constraint tangent L10 A0
  constraint tangent L5 A0
  constraint tangent L10 A1
  constraint tangent L11 A1
  constraint equal A0 A1
  constraint coincident P3 L11
  constraint coincident P3 L5
  constraint tangent L11 A2
  constraint tangent L5 A2
  constraint equal A0 A2
  constraint coincident P4 L12
  constraint coincident P4 L6
  constraint tangent L12 A3
  constraint tangent L6 A3
  constraint equal A0 A3
  constraint coincident P5 L6
  constraint coincident P5 L13
  constraint tangent L6 A4
  constraint tangent L13 A4
  constraint equal A0 A4
  constraint tangent L13 A5
  constraint tangent L12 A5
  constraint equal A0 A5
  constraint tangent L14 A6
  constraint tangent L15 A6
  constraint equal A0 A6
  constraint coincident P6 L14
  constraint coincident P6 L7
  constraint tangent L14 A7
  constraint tangent L7 A7
  constraint equal A0 A7
  constraint coincident P7 L7
  constraint coincident P7 L15
  constraint tangent L7 A8
  constraint tangent L15 A8
  constraint equal A0 A8
  constraint coincident P1 L8
  constraint coincident P1 L4
  constraint tangent L8 A9
  constraint tangent L4 A9
  constraint equal A0 A9
  constraint coincident P0 L9
  constraint coincident P0 L4
  constraint tangent L9 A10
  constraint tangent L4 A10
  constraint equal A0 A10
  constraint tangent L9 A11
  constraint tangent L8 A11
  measures "d93" distance of P0 P1
  measures "d94" distance of P4 P5
  measures "d95" distance of P6 P7
  measures "d96" distance of P2 P3
  measures "d97" horizontal distance of origin P1
  measures "d98" horizontal distance of origin P4
  measures "d99" vertical distance of origin P6
  measures "d100" vertical distance of origin P2
  measures "d101" distance of L3 L6
  measures "d102" distance of L0 L7
  measures "d103" distance of L2 L5
  measures "d104" distance of L1 L4
  measures "d105" radius of A0
  measures "d112" radius of A11
extrude "Extrude11" cut sketch "Sketch9" along normal blind 0 and the other way blind 6 contours L4 L8 L9 A9 A10 A11 | L5 L10 L11 A0 A1 A2 | L6 L12 L13 A3 A4 A5 | L7 L14 L15 A6 A7 A8 bodies 1
sketch "Sketch10" plane through (0, 22.5, 0) normal (0, -1, 0) x (1, 0, 0)
  circle A0 centre (0, 24.5) radius 12.5
  line L0 (26.575, 38.5) -> (-26.575, 38.5)
  line L1 (-26.575, 38.5) -> (-26.575, 1)
  line L2 (-26.575, 1) -> (26.575, 1)
  line L3 (26.575, 1) -> (26.575, 38.5)
  circle A1 centre (20, 18.5) radius 2.75
  circle A2 centre (-20, 30.5) radius 2.75
  circle A3 centre (20, 30.5) radius 2.75
  circle A4 centre (-20, 18.5) radius 2.75
  line L4 (-21.575, 9.5) -> (21.575, 9.5)
  line L5 (24.075, 7) -> (24.075, 6)
  line L6 (21.575, 3.5) -> (-21.575, 3.5)
  line L7 (-24.075, 6) -> (-24.075, 7)
  arc A5 (-21.575, 9.5) -> (-24.075, 7) centre (-21.575, 7) ccw
  arc A6 (-24.075, 6) -> (-21.575, 3.5) centre (-21.575, 6) ccw
  arc A7 (21.575, 3.5) -> (24.075, 6) centre (21.575, 6) ccw
  arc A8 (24.075, 7) -> (21.575, 9.5) centre (21.575, 7) ccw
  dimension "d113" = 2.5
  dimension "d114" = 2.5
  dimension "d115" = 2.5
  dimension "d116" = 15
  dimension "d117" = 2.5
  constraint horizontal L4
  constraint vertical L5
  constraint horizontal L6
  constraint vertical L7
  constraint tangent L4 A5
  constraint tangent L7 A5
  constraint tangent L7 A6
  constraint tangent L6 A6
  constraint equal A5 A6
  constraint tangent L6 A7
  constraint tangent L5 A7
  constraint equal A5 A7
  constraint tangent L5 A8
  constraint tangent L4 A8
  constraint equal A5 A8
  measures "d113" distance of L2 L6
  measures "d114" distance of L1 L7
  measures "d115" distance of L3 L5
  measures "d116" distance of A0.centre L4
  measures "d117" radius of A5
extrude "Extrude13" cut sketch "Sketch10" against normal blind 6 contours L4 L5 L6 L7 A5 A6 A7 A8 bodies 1
extrude "Extrude14" add 1 faces at (5.4657, 25.6667, -5) along direction (0, 0, -1) blind 5 on bodies 1 bodies 1
sketch "Sketch13" plane through (26.575, 0, 0) normal (1, 0, 0) x (0, 1, 0)
  line L0 (28.5, 38.5) -> (22.5, 38.5)
  line L1 (22.5, 38.5) -> (22.5, 1)
  line L2 (22.5, 1) -> (-22.5, 1)
  line L3 (-22.5, 1) -> (-22.5, -10)
  line L4 (-22.5, -10) -> (28.5, -10)
  line L5 (28.5, -10) -> (28.5, 38.5)
  line L6 (-13, -1.5) -> (13, -1.5)
  line L7 (15, -3.5) -> (15, -5.5)
  line L8 (13, -7.5) -> (-13, -7.5)
  line L9 (-15, -5.5) -> (-15, -3.5)
  arc A0 (-13, -1.5) -> (-15, -3.5) centre (-13, -3.5) ccw
  arc A1 (-15, -5.5) -> (-13, -7.5) centre (-13, -5.5) ccw
  arc A2 (13, -7.5) -> (15, -5.5) centre (13, -5.5) ccw
  arc A3 (15, -3.5) -> (13, -1.5) centre (13, -3.5) ccw
  dimension "d124" = 2.5
  dimension "d125" = 2.5
  dimension "d126" = 7.5
  dimension "d127" = 13.5
  dimension "d128" = 2
  constraint horizontal L6
  constraint vertical L7
  constraint horizontal L8
  constraint vertical L9
  constraint tangent L6 A0
  constraint tangent L9 A0
  constraint tangent L9 A1
  constraint tangent L8 A1
  constraint equal A0 A1
  constraint tangent L8 A2
  constraint tangent L7 A2
  constraint equal A0 A2
  constraint tangent L7 A3
  constraint tangent L6 A3
  constraint equal A0 A3
  measures "d124" distance of L2 L6
  measures "d125" distance of L4 L8
  measures "d126" distance of L3 L9
  measures "d127" distance of L5 L7
  measures "d128" radius of A0
extrude "Extrude15" cut sketch "Sketch13" against normal blind 4 contours L6 L7 L8 L9 A0 A1 A2 A3 bodies 1
sketch "Sketch14" plane through (0, -22.5, 0) normal (0, -1, 0) x (1, 0, 0)
  line L0 (26.575, -10) -> (26.575, 1)
  line L1 (26.575, 1) -> (-26.575, 1)
  line L2 (-26.575, 1) -> (-26.575, -10)
  line L3 (-26.575, -10) -> (26.575, -10)
  line L4 (-15.5, -1.5) -> (15.5, -1.5)
  line L5 (17.5, -3.5) -> (17.5, -5.5)
  line L6 (15.5, -7.5) -> (-15.5, -7.5)
  line L7 (-17.5, -5.5) -> (-17.5, -3.5)
  arc A0 (-15.5, -1.5) -> (-17.5, -3.5) centre (-15.5, -3.5) ccw
  arc A1 (-17.5, -5.5) -> (-15.5, -7.5) centre (-15.5, -5.5) ccw
  arc A2 (15.5, -7.5) -> (17.5, -5.5) centre (15.5, -5.5) ccw
  arc A3 (17.5, -3.5) -> (15.5, -1.5) centre (15.5, -3.5) ccw
  dimension "d131" = 2.5
  dimension "d132" = 2.5
  dimension "d133" = 9.075
  dimension "d134" = 9.075
  dimension "d135" = 2
  constraint horizontal L4
  constraint vertical L5
  constraint horizontal L6
  constraint vertical L7
  constraint tangent L4 A0
  constraint tangent L7 A0
  constraint tangent L7 A1
  constraint tangent L6 A1
  constraint equal A0 A1
  constraint tangent L6 A2
  constraint tangent L5 A2
  constraint equal A0 A2
  constraint tangent L4 A3
  constraint tangent L5 A3
  constraint equal A0 A3
  measures "d131" distance of L1 L4
  measures "d132" distance of L3 L6
  measures "d133" distance of L2 L7
  measures "d134" distance of L0 L5
  measures "d135" radius of A0
extrude "Extrude16" cut sketch "Sketch14" against normal blind 4 contours L4 L5 L6 L7 A0 A1 A2 A3 bodies 1
sketch "Sketch15" plane through (-26.575, 0, 0) normal (-1, 0, 0) x (0, -1, 0)
  line L0 (-22.5, 38.5) -> (-28.5, 38.5)
  line L1 (-28.5, 38.5) -> (-28.5, -10)
  line L2 (-28.5, -10) -> (22.5, -10)
  line L3 (22.5, -10) -> (22.5, 1)
  line L4 (22.5, 1) -> (-22.5, 1)
  line L5 (-22.5, 1) -> (-22.5, 38.5)
  line L6 (-13, -1.5) -> (13, -1.5)
  line L7 (15, -3.5) -> (15, -5.5)
  line L8 (13, -7.5) -> (-13, -7.5)
  line L9 (-15, -5.5) -> (-15, -3.5)
  arc A0 (15, -3.5) -> (13, -1.5) centre (13, -3.5) ccw
  arc A1 (13, -7.5) -> (15, -5.5) centre (13, -5.5) ccw
  arc A2 (-15, -5.5) -> (-13, -7.5) centre (-13, -5.5) ccw
  arc A3 (-13, -1.5) -> (-15, -3.5) centre (-13, -3.5) ccw
  dimension "d138" = 2.5
  dimension "d139" = 2.5
  dimension "d140" = 7.5
  dimension "d141" = 13.5
  dimension "d142" = 2
  constraint horizontal L6
  constraint vertical L7
  constraint horizontal L8
  constraint vertical L9
  constraint tangent L7 A0
  constraint tangent L6 A0
  constraint tangent L7 A1
  constraint tangent L8 A1
  constraint equal A0 A1
  constraint tangent L8 A2
  constraint tangent L9 A2
  constraint equal A0 A2
  constraint tangent L9 A3
  constraint tangent L6 A3
  constraint equal A0 A3
  measures "d138" distance of L4 L6
  measures "d139" distance of L2 L8
  measures "d140" distance of L3 L7
  measures "d141" distance of L1 L9
  measures "d142" radius of A0
extrude "Extrude17" cut sketch "Sketch15" against normal blind 4 contours L6 L7 L8 L9 A0 A1 A2 A3 bodies 1
sketch "Sketch16" plane through (0, 28.5, 0) normal (0, 1, 0) x (-1, 0, 0)
  line L0 (-24.075, 6) -> (-24.075, 7)
  arc A0 (-21.575, 9.5) -> (-24.075, 7) centre (-21.575, 7) ccw
  line L1 (-21.575, 9.5) -> (21.575, 9.5)
  arc A1 (24.075, 7) -> (21.575, 9.5) centre (21.575, 7) ccw
  line L2 (24.075, 7) -> (24.075, 6)
  arc A2 (21.575, 3.5) -> (24.075, 6) centre (21.575, 6) ccw
  line L3 (21.575, 3.5) -> (-21.575, 3.5)
  arc A3 (-24.075, 6) -> (-21.575, 3.5) centre (-21.575, 6) ccw
  circle A4 centre (0, 24.5) radius 12.5
  line L4 (26.575, 38.5) -> (-26.575, 38.5)
  line L5 (-26.575, 38.5) -> (-26.575, -10)
  line L6 (-26.575, -10) -> (26.575, -10)
  line L7 (26.575, -10) -> (26.575, 38.5)
  circle A5 centre (20, 18.5) radius 5
  circle A6 centre (-20, 30.5) radius 5
  circle A7 centre (20, 30.5) radius 5
  circle A8 centre (-20, 18.5) radius 5
  line L8 (-15.5, -1.5) -> (15.5, -1.5)
  line L9 (17.5, -3.5) -> (17.5, -5.5)
  line L10 (15.5, -7.5) -> (-15.5, -7.5)
  line L11 (-17.5, -5.5) -> (-17.5, -3.5)
  arc A9 (-15.5, -1.5) -> (-17.5, -3.5) centre (-15.5, -3.5) ccw
  arc A10 (-17.5, -5.5) -> (-15.5, -7.5) centre (-15.5, -5.5) ccw
  arc A11 (15.5, -7.5) -> (17.5, -5.5) centre (15.5, -5.5) ccw
  arc A12 (17.5, -3.5) -> (15.5, -1.5) centre (15.5, -3.5) ccw
  dimension "d145" = 5
  dimension "d146" = 2.5
  dimension "d147" = 9.075
  dimension "d148" = 9.075
  dimension "d149" = 2
  constraint horizontal L8
  constraint vertical L9
  constraint horizontal L10
  constraint vertical L11
  constraint tangent L8 A9
  constraint tangent L11 A9
  constraint tangent L11 A10
  constraint tangent L10 A10
  constraint equal A9 A10
  constraint tangent L10 A11
  constraint tangent L9 A11
  constraint equal A9 A11
  constraint tangent L9 A12
  constraint tangent L8 A12
  constraint equal A9 A12
  measures "d145" distance of L3 L8
  measures "d146" distance of L6 L10
  measures "d147" distance of L5 L11
  measures "d148" distance of L7 L9
  measures "d149" radius of A9
extrude "Extrude18" cut sketch "Sketch16" against normal blind 10 contours L8 L9 L10 L11 A9 A10 A11 A12 bodies 1
equation "d7 = ( 2.25 in / 2 )"
equation "d8 = ( 45 / 2 ) * 1 mm"
equation "d31 = ( 2.25 in - 40 mm ) / 2"
equation "d127 = 7.5 mm + 6 mm"
equation "d133 = ( ( 53.15 - 35 ) / 2 ) * 1 mm"
equation "d134 = ( ( 53.15 - 35 ) / 2 ) * 1 mm"

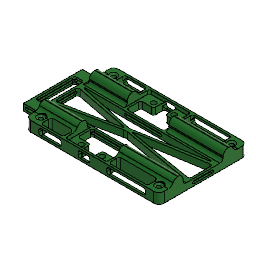
design "TM Foundation"
Autodesk Fusion 360 part; units mm, degrees
sketch "Sketch1" plane through (0, 0, 0) normal (0, 0, 1) x (1, 0, 0)
  line L0 (-72.5, 28.55) -> (72.5, 28.55)
  line L1 (72.5, 28.55) -> (72.5, -28.55)
  line L2 (72.5, -28.55) -> (-72.5, -28.55)
  line L3 (-72.5, -28.55) -> (-72.5, 28.55)
  dimension "d1" = 145
  dimension "d2" = 72.5
  dimension "d3" = 57.1
  dimension "d4" = 28.55
  constraint horizontal L0
  constraint vertical L1
  constraint horizontal L2
  constraint vertical L3
  measures "d1" distance of L1 L3
  measures "d2" distance of origin L1
  measures "d3" distance of L0 L2
  measures "d4" distance of origin L0
extrude "Extrude1" add sketch "Sketch1" along normal blind 6.5
ref_plane "WorkPlane1" through (-62.5, 0, 3.25) normal (-1, 0, 0) x (0, -1, 0)
sketch "Sketch6" plane through (-62.5, 0, 0) normal (-1, 0, 0) x (0, -1, 0)
  line L0 (-28.55, 6.5) -> (-28.55, 15.75)
  line L1 (-28.55, 15.75) -> (-24.3, 15.75)
  line L2 (-16.3, 6.5) -> (16.3, 6.5)
  line L3 (28.55, 6.5) -> (28.55, 15.75)
  line L4 (28.55, 15.75) -> (24.3, 15.75)
  line L5 (-19.3, 10.75) -> (-19.3, 9.5)
  line L6 (19.3, 10.75) -> (19.3, 9.5)
  arc A0 (-19.3, 9.5) -> (-16.3, 6.5) centre (-16.3, 9.5) ccw
  arc A1 (16.3, 6.5) -> (19.3, 9.5) centre (16.3, 9.5) ccw
  arc A2 (-19.3, 10.75) -> (-24.3, 15.75) centre (-24.3, 10.75) ccw
  arc A3 (24.3, 15.75) -> (19.3, 10.75) centre (24.3, 10.75) ccw
  line L7 (-28.55, 6.5) -> (28.55, 6.5)
  point P0 (-19.3, 15.75)
  point P1 (-28.55, 0)
  point P2 (-28.55, 6.5)
  point P3 (-28.55, 6.5)
  point P4 (19.3, 15.75)
  dimension "d36" = 9.25
  dimension "d37" = 9.25
  dimension "d38" = 57.1
  dimension "d39" = 9.25
  dimension "d40" = 9.25
  dimension "d41" = 3
  dimension "d42" = 5
  constraint vertical L0
  constraint perpendicular L0 L1
  constraint vertical P3 P1
  constraint coincident P3 P2
  constraint perpendicular L0 L2
  constraint perpendicular L2 L3
  constraint perpendicular L3 L4
  constraint perpendicular L2 L5
  constraint perpendicular L2 L6
  constraint coincident P3 L2
  constraint tangent L5 A0
  constraint tangent L2 A0
  constraint coincident L3.start L2
  constraint tangent L2 A1
  constraint tangent L6 A1
  constraint equal A0 A1
  constraint coincident P0 L1
  constraint coincident P0 L5
  constraint tangent L1 A2
  constraint tangent L5 A2
  constraint coincident P4 L6
  constraint coincident P4 L4
  constraint tangent L6 A3
  constraint tangent L4 A3
  constraint equal A2 A3
  measures "d36" distance of P3 L0.end
  measures "d37" distance of L0.end P0
  measures "d38" distance of P3 L3.start
  measures "d39" distance of L3.start L3.end
  measures "d40" distance of L3.end P4
  measures "d41" radius of A0
  measures "d42" radius of A2